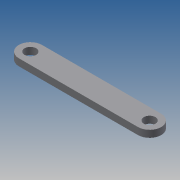
# Autodesk Inventor part: 02連桿25
Saved by Autodesk Inventor 2015 (Build 190159000, 159)
## iProperties
Created: 2017-12-26
Part Number: 02連桿25
Material: 一般
Document SubType Name: Modeling
Designer: user
Density: 1 g/cm^3
Appearance: 預設
Author: user
Autodesk Inventor part; units mm, degrees
ref_plane "YZ Plane" through (0, 0, 0) normal (1, 0, 0) x (0, 1, 0)
ref_plane "XZ Plane" through (0, 0, 0) normal (0, 1, 0) x (-1, 0, 0)
ref_plane "XY Plane" through (0, 0, 0) normal (0, 0, 1) x (1, 0, 0)
sketch "草圖1" plane through (0, 0, 0) normal (0, 0, 1) x (1, 0, 0)
  line L0 (0, 0) -> (51.5, 0) construction
  line L1 (0, -5) -> (51.5, -5)
  line L2 (51.5, 5) -> (0, 5)
  arc A0 (0, 5) -> (0, -5) centre (0, 0) ccw
  arc A1 (51.5, -5) -> (51.5, 5) centre (51.5, 0) ccw
  point P0 (25.75, 0)
  dimension "d0" = 51.5
  dimension "d1" = 5
  constraints: 8 end point, 4 point on circle, 4 tangent, 2 centre point, 1 horizontal, 1 midpoint, 1 parallel
  measures "d0" distance of L1.start L1.end
  measures "d1" radius of A1
extrude "擠出1" add sketch "草圖1" along normal blind 3
hole "孔1" at (51.5, 0, 3) direction (0, 0, -1) diameter 5 depth 8 tip angle 118
hole "孔2" at (0, 0, 3) direction (0, 0, -1) diameter 5 depth 8 tip angle 118
